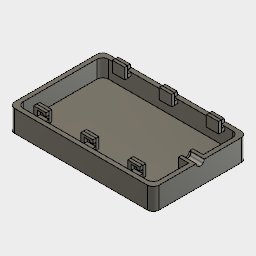
LED_Light_Case_Top v6 (Autodesk Fusion 360 design; units mm, degrees)
Autodesk Fusion 360 part; units mm, degrees
sketch "Sketch1" plane through (0, 0, 0) normal (0, 1, 0) x (1, 0, 0)
  line L0 (4, 0) -> (96, 0)
  line L1 (100, 4) -> (100, 61)
  line L2 (96, 65) -> (4, 65)
  line L3 (0, 61) -> (0, 4)
  line L4 (93, 62) -> (7, 62)
  line L5 (3, 58) -> (3, 7)
  line L6 (7, 3) -> (93, 3)
  line L7 (97, 7) -> (97, 58)
  arc A0 (3, 7) -> (7, 3) centre (7, 7) ccw
  arc A1 (93, 3) -> (97, 7) centre (93, 7) ccw
  arc A2 (97, 58) -> (93, 62) centre (93, 58) ccw
  arc A3 (7, 62) -> (3, 58) centre (7, 58) ccw
  arc A4 (4, 65) -> (0, 61) centre (4, 61) ccw
  arc A5 (0, 4) -> (4, 0) centre (4, 4) ccw
  arc A6 (96, 0) -> (100, 4) centre (96, 4) ccw
  arc A7 (100, 61) -> (96, 65) centre (96, 61) ccw
  point P0 (100, 0)
  point P1 (0, 65)
  dimension "d1" = 100
  dimension "d2" = 65
  dimension "d4" = 4
  measures "d1" distance of origin P0
  measures "d2" distance of origin P1
  measures "d4" radius of A0
extrude "Extrude1" add sketch "Sketch1" along normal blind 3 contours L4 L5 L6 L7 A0 A1 A2 A3 makes body 1
extrude "Extrude2" add sketch "Sketch1" along normal blind 15 bodies 1
sketch "Sketch3" plane through (0, 3, 0) normal (0, 1, 0) x (-1, 0, 0)
  arc A0 (-7, -62) -> (-3, -58) centre (-7, -58) ccw
  line L0 (-3, -58) -> (-3, -7)
  arc A1 (-3, -7) -> (-7, -3) centre (-7, -7) ccw
  line L1 (-7, -3) -> (-93, -3)
  arc A2 (-93, -3) -> (-97, -7) centre (-93, -7) ccw
  line L2 (-97, -7) -> (-97, -58)
  arc A3 (-97, -58) -> (-93, -62) centre (-93, -58) ccw
  line L3 (-93, -62) -> (-7, -62)
  line L4 (-97, -37.5) -> (-90, -37.5)
  line L5 (-90, -37.5) -> (-90, -27.5)
  line L6 (-90, -27.5) -> (-97, -27.5)
  line L7 (-97, -27.5) -> (-97, -37.5)
  line L8 (-93, -62) -> (-7, -62)
  dimension "d9" = 24.5
  dimension "d10" = 10
  dimension "d11" = 7
  measures "d9" distance of L4 L8
  measures "d10" distance of L4.end L5.end
  measures "d11" distance of L5.end L6.end
extrude "Extrude3" add sketch "Sketch3" along normal blind 12 contours L2 L4 L5 L6 L7 bodies 1
sketch "Sketch4" plane through (90, 0, 0) normal (-1, 0, 0) x (0, 0, 1)
  line L0 (-37.5, 3) -> (-27.5, 3)
  line L1 (-27.5, 3) -> (-27.5, 15)
  line L2 (-27.5, 15) -> (-37.5, 15)
  line L3 (-37.5, 15) -> (-37.5, 3)
  circle A0 centre (-32.5, 15) radius 2.5
  dimension "d14" = 5
  measures "d14" diameter of A0
extrude "Extrude4" cut sketch "Sketch4" against normal blind 10 contours L2 A0 picked at (-31.8726, 13.6334) bodies 1
sketch "Sketch5" plane through (90, 0, 0) normal (-1, 0, 0) x (0, 0, 1)
  arc A0 (-35, 15) -> (-30, 15) centre (-32.5, 15) ccw
  line L0 (-35, 15) -> (-37.5, 15)
  line L1 (-37.5, 15) -> (-37.5, 3)
  line L2 (-37.5, 3) -> (-27.5, 3)
  line L3 (-27.5, 3) -> (-27.5, 15)
  line L4 (-27.5, 15) -> (-30, 15)
  circle A1 centre (-32.5, 15) radius 2.8
  dimension "d17" = 5.6
  measures "d17" diameter of A1
extrude "Extrude5" cut sketch "Sketch5" against normal blind 9 from surface at -1 contours A0 L0 L4 A1 picked at (-29.8197, 14.7367) bodies 1
sketch "Sketch6" plane through (0, 0, -62) normal (0, 0, 1) x (1, 0, 0)
  line L0 (7, 3) -> (93, 3)
  line L1 (93, 3) -> (93, 15)
  line L2 (93, 15) -> (7, 15)
  line L3 (7, 15) -> (7, 3)
  line L4 (14, 15) -> (16.5, 15)
  line L5 (16.5, 15) -> (16.5, 20)
  line L6 (16.5, 20) -> (14, 20)
  line L7 (14, 20) -> (14, 15)
  line L8 (16.5, 20) -> (22.5, 20)
  line L9 (22.5, 20) -> (22.5, 18.5)
  line L10 (22.5, 18.5) -> (16.5, 18.5)
  line L11 (16.5, 18.5) -> (16.5, 20)
  line L12 (22.5, 18.5) -> (20.25, 18.5)
  line L13 (20.25, 18.5) -> (20.25, 17.5)
  line L14 (20.25, 17.5) -> (22.5, 17.5)
  line L15 (22.5, 17.5) -> (22.5, 18.5)
  line L16 (14, 15) -> (16.5, 15)
  line L17 (16.5, 15) -> (16.5, 12.5)
  line L18 (16.5, 12.5) -> (14, 12.5)
  line L19 (14, 12.5) -> (14, 15)
  line L20 (16.5, 12.5) -> (22.5, 12.5)
  line L21 (22.5, 12.5) -> (22.5, 15)
  line L22 (22.5, 15) -> (16.5, 15)
  line L23 (16.5, 15) -> (16.5, 12.5)
  line L24 (22.5, 12.5) -> (14, 12.5)
  line L25 (14, 12.5) -> (14, 20)
  line L26 (14, 20) -> (22.5, 20)
  line L27 (22.5, 20) -> (22.5, 12.5)
  line L28 (46.5, 15) -> (49, 15)
  line L29 (46.5, 20) -> (55, 20)
  line L30 (46.5, 15) -> (49, 15)
  line L31 (55, 17.5) -> (55, 18.5)
  line L32 (52.75, 17.5) -> (55, 17.5)
  line L33 (52.75, 18.5) -> (52.75, 17.5)
  line L34 (55, 12.5) -> (55, 15)
  line L35 (49, 12.5) -> (46.5, 12.5)
  line L36 (49, 15) -> (49, 12.5)
  line L37 (49, 20) -> (46.5, 20)
  line L38 (49, 15) -> (49, 20)
  line L39 (49, 12.5) -> (55, 12.5)
  line L40 (46.5, 12.5) -> (46.5, 15)
  line L41 (49, 20) -> (55, 20)
  line L42 (46.5, 20) -> (46.5, 15)
  line L43 (55, 18.5) -> (52.75, 18.5)
  line L44 (49, 18.5) -> (49, 20)
  line L45 (55, 18.5) -> (49, 18.5)
  line L46 (55, 20) -> (55, 18.5)
  line L47 (55, 12.5) -> (46.5, 12.5)
  line L48 (49, 15) -> (49, 12.5)
  line L49 (55, 15) -> (49, 15)
  line L50 (55, 20) -> (55, 12.5)
  line L51 (46.5, 12.5) -> (46.5, 20)
  line L52 (55, 20) -> (55, 12.5)
  line L53 (55, 15) -> (49, 15)
  line L54 (49, 18.5) -> (49, 20)
  line L55 (55, 12.5) -> (46.5, 12.5)
  line L56 (46.5, 20) -> (46.5, 15)
  line L57 (46.5, 12.5) -> (46.5, 15)
  line L58 (55, 18.5) -> (52.75, 18.5)
  line L59 (55, 18.5) -> (49, 18.5)
  line L60 (49, 15) -> (49, 20)
  line L61 (49, 20) -> (55, 20)
  line L62 (49, 15) -> (49, 12.5)
  line L63 (49, 12.5) -> (55, 12.5)
  line L64 (55, 12.5) -> (55, 15)
  line L65 (49, 20) -> (46.5, 20)
  line L66 (52.75, 17.5) -> (55, 17.5)
  line L67 (49, 12.5) -> (46.5, 12.5)
  line L68 (52.75, 18.5) -> (52.75, 17.5)
  line L69 (46.5, 15) -> (49, 15)
  line L70 (46.5, 15) -> (49, 15)
  line L71 (55, 17.5) -> (55, 18.5)
  line L72 (46.5, 20) -> (55, 20)
  line L73 (46.5, 12.5) -> (46.5, 20)
  line L74 (49, 15) -> (49, 12.5)
  line L75 (55, 20) -> (55, 18.5)
  line L76 (79, 12.5) -> (79, 20)
  line L77 (81.5, 15) -> (81.5, 20)
  line L78 (87.5, 20) -> (87.5, 12.5)
  line L79 (79, 20) -> (79, 15)
  line L80 (79, 12.5) -> (79, 20)
  line L81 (87.5, 20) -> (87.5, 12.5)
  line L82 (79, 20) -> (87.5, 20)
  line L83 (79, 20) -> (79, 15)
  line L84 (81.5, 12.5) -> (79, 12.5)
  line L85 (87.5, 17.5) -> (87.5, 18.5)
  line L86 (81.5, 12.5) -> (87.5, 12.5)
  line L87 (85.25, 18.5) -> (85.25, 17.5)
  line L88 (81.5, 20) -> (79, 20)
  line L89 (81.5, 15) -> (81.5, 20)
  line L90 (85.25, 17.5) -> (87.5, 17.5)
  line L91 (87.5, 12.5) -> (79, 12.5)
  line L92 (87.5, 15) -> (81.5, 15)
  line L93 (87.5, 15) -> (81.5, 15)
  line L94 (79, 15) -> (81.5, 15)
  line L95 (79, 15) -> (81.5, 15)
  line L96 (87.5, 12.5) -> (87.5, 15)
  line L97 (81.5, 20) -> (87.5, 20)
  line L98 (87.5, 12.5) -> (79, 12.5)
  line L99 (87.5, 18.5) -> (85.25, 18.5)
  line L100 (81.5, 18.5) -> (81.5, 20)
  line L101 (87.5, 18.5) -> (81.5, 18.5)
  line L102 (87.5, 20) -> (87.5, 18.5)
  line L103 (81.5, 18.5) -> (81.5, 20)
  line L104 (87.5, 18.5) -> (85.25, 18.5)
  line L105 (81.5, 15) -> (81.5, 12.5)
  line L106 (79, 12.5) -> (79, 15)
  line L107 (87.5, 18.5) -> (81.5, 18.5)
  line L108 (81.5, 12.5) -> (87.5, 12.5)
  line L109 (81.5, 20) -> (87.5, 20)
  line L110 (79, 12.5) -> (79, 15)
  line L111 (85.25, 17.5) -> (87.5, 17.5)
  line L112 (85.25, 18.5) -> (85.25, 17.5)
  line L113 (81.5, 12.5) -> (79, 12.5)
  line L114 (81.5, 15) -> (81.5, 12.5)
  line L115 (81.5, 20) -> (79, 20)
  line L116 (81.5, 15) -> (81.5, 12.5)
  line L117 (79, 15) -> (81.5, 15)
  line L118 (79, 20) -> (87.5, 20)
  line L119 (87.5, 12.5) -> (87.5, 15)
  line L120 (79, 15) -> (81.5, 15)
  line L121 (87.5, 17.5) -> (87.5, 18.5)
  line L122 (81.5, 15) -> (81.5, 12.5)
  line L123 (87.5, 20) -> (87.5, 18.5)
  dimension "d21" = 7
  dimension "d22" = 2.5
  dimension "d23" = 5
  dimension "d24" = 1.5
  dimension "d25" = 1
  dimension "d26" = 3.75
  dimension "d27" = 6
  dimension "d30" = 2.5
  dimension "d47" = 6
  dimension "d56" = 2.5
  dimension "d57" = 5
  dimension "d58" = 1.5
  dimension "d59" = 1
  dimension "d60" = 3.75
  dimension "d61" = 6
  dimension "d62" = 2.5
  dimension "d63" = 6
  dimension "d64" = 2.5
  dimension "d65" = 5
  dimension "d66" = 1.5
  dimension "d67" = 1
  dimension "d68" = 3.75
  dimension "d69" = 6
  dimension "d70" = 2.5
  dimension "d71" = 6
  dimension "d72" = 2.5
  dimension "d73" = 5
  dimension "d74" = 1.5
  dimension "d75" = 1
  dimension "d76" = 3.75
  dimension "d77" = 6
  dimension "d78" = 2.5
  dimension "d79" = 6
  dimension "d80" = 2.5
  dimension "d81" = 5
  dimension "d82" = 1.5
  dimension "d83" = 1
  dimension "d84" = 3.75
  dimension "d85" = 6
  dimension "d86" = 2.5
  dimension "d87" = 6
  measures "d21" distance of L3 L7
  measures "d22" distance of L5.end L6.end
  measures "d23" distance of L4.start L6.end
  measures "d24" distance of L5.end L10.end
  measures "d25" distance of L9.end L14.end
  measures "d26" distance of L5 L13
  measures "d27" distance of L5.end L8.end
  measures "d30" distance of L4.start L18.end
  measures "d47" distance of L17.end L20.end
  measures "d56" distance of L37.start L29.start
  measures "d57" distance of L28.start L29.start
  measures "d58" distance of L44.start L37.start
  measures "d59" distance of L31.end L31.start
  measures "d60" distance of L33 L38
  measures "d61" distance of L29.end L37.start
  measures "d62" distance of L35.end L28.start
  measures "d63" distance of L34.start L35.start
  measures "d64" distance of L37.start L29.start
  measures "d65" distance of L29.start L28.start
  measures "d66" distance of L44.start L37.start
  measures "d67" distance of L31.end L31.start
  measures "d68" distance of L60 L68
  measures "d69" distance of L37.start L29.end
  measures "d70" distance of L28.start L35.end
  measures "d71" distance of L34.start L35.start
  measures "d72" distance of L77.end L76.end
  measures "d73" distance of L76.end L79.end
  measures "d74" distance of L100.start L77.end
  measures "d75" distance of L85.end L85.start
  measures "d76" distance of L87 L89
  measures "d77" distance of L77.end L78.start
  measures "d78" distance of L79.end L76.start
  measures "d79" distance of L78.end L84.start
  measures "d80" distance of L76.end L77.end
  measures "d81" distance of L79.end L76.end
  measures "d82" distance of L100.start L77.end
  measures "d83" distance of L85.end L85.start
  measures "d84" distance of L77 L112
  measures "d85" distance of L78.start L77.end
  measures "d86" distance of L79.end L76.start
  measures "d87" distance of L78.end L84.start
extrude "Extrude19" add sketch "Sketch6" along normal blind 2 from surface at 2.3 separate body contours L2 L78 L81 L86 L91 L92 L93 L96 L98 L105 L108 L114 L116 L119 L122 | L2 L77 L78 L81 L87 L89 L90 L92 L93 L101 L107 L111 L112 | L2 L76 L80 L84 L91 L94 L95 L98 L105 L106 L110 L113 L114 L116 L117 L120 L122 | L2 L76 L77 L79 L80 L82 L83 L88 L89 L94 L95 L100 L103 L115 L117 L118 L120 | L78 L81 L85 L87 L90 L99 L101 L104 L107 L111 L112 L121 | L77 L78 L81 L82 L89 L97 L99 L100 L101 L102 L103 L104 L107 L109 L118 L123 makes body 2
extrude "Extrude18" add sketch "Sketch6" along normal blind 2.3 separate body contours L2 L78 L81 L86 L91 L92 L93 L96 L98 L105 L108 L114 L116 L119 L122 makes body 3
extrude "Extrude16" add sketch "Sketch6" along normal blind 2 from surface at 2.3 separate body contours L2 L28 L29 L30 L37 L38 L42 L44 L51 L54 L56 L60 L65 L69 L70 L72 L73 | L2 L28 L30 L35 L36 L40 L47 L48 L51 L55 L57 L62 L67 L69 L70 L73 L74 | L2 L34 L36 L39 L47 L48 L49 L50 L52 L53 L55 L62 L63 L64 L74 | L2 L32 L33 L38 L45 L49 L50 L52 L53 L59 L60 L66 L68 | L31 L32 L33 L43 L45 L50 L52 L58 L59 L66 L68 L71 | L29 L38 L41 L43 L44 L45 L46 L50 L52 L54 L58 L59 L60 L61 L72 L75 makes body 4
extrude "Extrude15" add sketch "Sketch6" along normal blind 2.3 separate body contours L2 L34 L36 L39 L47 L48 L49 L50 L52 L53 L55 L62 L63 L64 L74 makes body 5
extrude "Extrude14" add sketch "Sketch6" along normal blind 2 from surface at 0.3 separate body contours L2 L28 L29 L30 L37 L38 L42 L44 L51 L54 L56 L60 L65 L69 L70 L72 L73 | L2 L28 L30 L35 L36 L40 L47 L48 L51 L55 L57 L62 L67 L69 L70 L73 L74 | L31 L32 L33 L43 L45 L50 L52 L58 L59 L66 L68 L71 | L29 L38 L41 L43 L44 L45 L46 L50 L52 L54 L58 L59 L60 L61 L72 L75 makes body 6
extrude "Extrude12" add sketch "Sketch6" along normal blind 2.3 separate body contours L2 L17 L20 L21 L22 L23 L24 L27 makes body 7
extrude "Extrude11" add sketch "Sketch6" along normal blind 2 from surface at 2.3 separate body contours L2 L4 L5 L6 L7 L11 L16 L25 L26 | L2 L4 L16 L17 L18 L19 L23 L24 L25 | L2 L5 L10 L13 L14 L22 L27 | L2 L17 L20 L21 L22 L23 L24 L27 | L5 L8 L9 L10 L11 L12 L26 L27 | L10 L12 L13 L14 L15 L27 makes body 8
sketch "Sketch7" plane through (0, 3, 0) normal (0, 1, 0) x (-1, 0, 0)
  line L0 (-97, -27.5) -> (-90, -27.5)
  line L1 (-90, -27.5) -> (-90, -37.5)
  line L2 (-90, -37.5) -> (-97, -37.5)
  line L3 (-97, -37.5) -> (-97, -58)
  arc A0 (-97, -58) -> (-93, -62) centre (-93, -58) ccw
  line L4 (-93, -62) -> (-7, -62)
  arc A1 (-7, -62) -> (-3, -58) centre (-7, -58) ccw
  line L5 (-3, -58) -> (-3, -7)
  arc A2 (-3, -7) -> (-7, -3) centre (-7, -7) ccw
  line L6 (-7, -3) -> (-93, -3)
  arc A3 (-93, -3) -> (-97, -7) centre (-93, -7) ccw
  line L7 (-97, -7) -> (-97, -27.5)
  line L8 (-90, -37.5) -> (-89, -37.5)
  line L9 (-89, -37.5) -> (-89, -32.5)
  line L10 (-89, -32.5) -> (-90, -32.5)
  line L11 (-90, -32.5) -> (-90, -37.5)
  dimension "d39" = 5
  dimension "d40" = 1
  measures "d39" distance of L1.end L10.end
  measures "d40" distance of L1.end L8.end
extrude "Extrude13" add sketch "Sketch6" along normal blind 2 from surface at 0.3 separate body contours L2 L4 L5 L6 L7 L11 L16 L25 L26 | L2 L4 L16 L17 L18 L19 L23 L24 L25 | L5 L8 L9 L10 L11 L12 L26 L27 | L10 L12 L13 L14 L15 L27 makes body 9
extrude "Extrude17" add sketch "Sketch6" along normal blind 2 from surface at 0.3 separate body contours L2 L76 L80 L84 L91 L94 L95 L98 L105 L106 L110 L113 L114 L116 L117 L120 L122 | L2 L76 L77 L79 L80 L82 L83 L88 L89 L94 L95 L100 L103 L115 L117 L118 L120 | L78 L81 L85 L87 L90 L99 L101 L104 L107 L111 L112 L121 | L77 L78 L81 L82 L89 L97 L99 L100 L101 L102 L103 L104 L107 L109 L118 L123 makes body 10
sketch "Sketch8" plane through (0, 3, 0) normal (0, 1, 0) x (-1, 0, 0)
  line L0 (-97, -27.5) -> (-90, -27.5)
  line L1 (-90, -27.5) -> (-90, -37.5)
  line L2 (-90, -37.5) -> (-97, -37.5)
  line L3 (-97, -37.5) -> (-97, -58)
  arc A0 (-97, -58) -> (-93, -62) centre (-93, -58) ccw
  line L4 (-93, -62) -> (-7, -62)
  arc A1 (-7, -62) -> (-3, -58) centre (-7, -58) ccw
  line L5 (-3, -58) -> (-3, -7)
  arc A2 (-3, -7) -> (-7, -3) centre (-7, -7) ccw
  line L6 (-7, -3) -> (-93, -3)
  arc A3 (-93, -3) -> (-97, -7) centre (-93, -7) ccw
  line L7 (-97, -7) -> (-97, -27.5)
  line L8 (-90, -37.5) -> (-89, -37.5)
  line L9 (-89, -37.5) -> (-89, -32.5)
  line L10 (-89, -32.5) -> (-90, -32.5)
  line L11 (-90, -32.5) -> (-90, -37.5)
  dimension "d104" = 5
  dimension "d105" = 1
  measures "d104" distance of L1.end L10.end
  measures "d105" distance of L1.end L8.end
extrude "Extrude20" add sketch "Sketch8" along normal blind 1 contours L1 L8 L9 L10 L11 bodies 1
mirror "Mirror2" about plane through (89, 3, -32.5) normal (0, 0, 1) of bodies 8 9 7 4 6 5 2 10 3 makes body 11 at (83.5, 15.8333, -5.3) makes body 12 at (83.5, 14.1667, -3) makes body 13 at (51, 15.8333, -5.3) makes body 14 at (51, 14.1667, -3) makes body 15 at (47.3333, 17.8333, -3.3) makes body 16 at (20.5, 14.1667, -3) makes body 17 at (18.5, 15.8333, -5.3) makes body 18 at (14.8333, 17.8333, -3.3) makes body 19 at (79.8333, 17.8333, -3.3)
